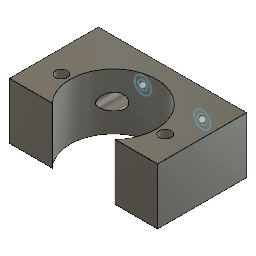
Erasing Motor Mount (Autodesk Fusion 360 design; units mm, degrees)
Autodesk Fusion 360 part; units mm, degrees
note: some values were not read from the file. Set by a fixed rule: which sketch regions a step uses.
sketch "Sketch1" plane through (0, 0, 0) normal (0, 0, 1) x (1, 0, 0)
  line L0 (25, 9.5) -> (-25, 9.5)
  line L1 (-25, 9.5) -> (-25, -9.5)
  line L2 (-25, -9.5) -> (25, -9.5)
  line L3 (25, -9.5) -> (25, 9.5)
  line L4 (25, 9.5) -> (-25, -9.5) construction
  line L5 (-25, 9.5) -> (25, -9.5) construction
  line L6 (60, -9.5) -> (110, -9.5)
  line L7 (110, -9.5) -> (110, 9.5)
  line L8 (110, 9.5) -> (60, 9.5)
  line L9 (60, 9.5) -> (60, -9.5)
  line L10 (60, -9.5) -> (110, 9.5) construction
  line L11 (110, -9.5) -> (60, 9.5) construction
  circle A0 centre (75, 0) radius 2
  circle A1 centre (95, 0) radius 2
  point P0 (85, 0)
  dimension "d1" = 50
  dimension "d2" = 19
  dimension "d22" = 50
  dimension "d23" = 19
  dimension "d26" = 4
  dimension "d27" = 4
  constraint perpendicular L0 L1
  constraint parallel L0 L2
  constraint parallel L1 L3
  constraint horizontal L0
  constraint coincident L4 origin
  constraint coincident L5 origin
  constraint perpendicular L6 L7
  constraint parallel L6 L8
  constraint parallel L7 L9
  constraint horizontal L6
  constraint coincident L10 P0
  constraint coincident L11 P0
  measures "d1" distance of L1.end L2.end
  measures "d2" distance of L0.end L1.end
  measures "d22" distance of L7.end L8.end
  measures "d23" distance of L6.end L7.end
  measures "d26" diameter of A0
  measures "d27" diameter of A1
extrude "Extrude1" add sketch "Sketch1" along normal blind 30 contours L0 L1 L2 L3
sketch "Sketch2" plane through (0, -9.5, 0) normal (0, -1, 0) x (1, 0, 0)
  line L0 (-25, 0) -> (25, 0)
  line L1 (25, 0) -> (25, 30)
  line L2 (25, 30) -> (-25, 30)
  line L3 (-25, 30) -> (-25, 0)
  circle A0 centre (0.0655, 20) radius 14.5
  line L4 (-40, 20) -> (55, 20)
  circle A1 centre (17.5655, 20) radius 2
  circle A2 centre (-17.4345, 20) radius 2
  dimension "d5" = 29
  dimension "d10" = 4
  dimension "d11" = 17.5
  dimension "d12" = 4
  dimension "d13" = 17.5
  constraint perpendicular L1 L4
  constraint coincident L4 A1.centre
  constraint coincident L4 A2.centre
  measures "d5" diameter of A0
  measures "d10" diameter of A1
  measures "d11" distance of A0.centre A1.centre
  measures "d12" diameter of A2
  measures "d13" distance of A0.centre A2.centre
extrude "Extrude2" cut sketch "Sketch2" against normal blind 19 contours L4 A2 | L4 A2 | L4 A1 | L4 A1 | L2 A0 L4 | A0 L4
sketch "Sketch3" plane through (0, 0, 0) normal (0, 0, -1) x (-1, 0, 0)
  line L0 (-25, 9.5) -> (-25, -9.5)
  line L1 (-25, -9.5) -> (25, -9.5)
  line L2 (25, -9.5) -> (25, 9.5)
  line L3 (25, 9.5) -> (-25, 9.5)
  circle A0 centre (-10, 0) radius 1.5
  circle A1 centre (-10, 0) radius 2.75
  circle A2 centre (10, 0) radius 1.5
  circle A3 centre (10, 0) radius 2.75
  dimension "d14" = 3
  dimension "d15" = 5.5
  dimension "d16" = 3
  dimension "d17" = 5.5
  constraint concentric A0 A1
  constraint concentric A2 A3
  measures "d14" diameter of A0
  measures "d15" diameter of A1
  measures "d16" diameter of A2
  measures "d17" diameter of A3
extrude "Extrude3" cut sketch "Sketch3" against normal blind 15 contours A0 | A1 | A2 | A3
extrude "Extrude4" add sketch "Sketch3" against normal blind 3 contours A1 | A3
